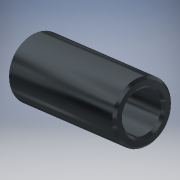
# Autodesk Inventor part: Component 31(Rod Axle)
Saved by Autodesk Inventor 2018 (Build 220112000, 112)
## iProperties
Created: 2023-04-01
Part Number: Component 31(Rod Axle)
Material: Generic
Document SubType Name: Modeling
Designer: Habib Mohamed
Density: 1 g/cm^3
Appearance: Iron Gray
Author: Habib Mohamed
Autodesk Inventor part; units mm, degrees
ref_plane "YZ Plane" through (0, 0, 0) normal (1, 0, 0) x (0, 1, 0)
ref_plane "XZ Plane" through (0, 0, 0) normal (0, 1, 0) x (-1, 0, 0)
ref_plane "XY Plane" through (0, 0, 0) normal (0, 0, 1) x (1, 0, 0)
sketch "Sketch1" plane through (0, 0, 0) normal (1, 0, 0) x (0, 1, 0)
  circle A0 centre (0, 0) radius 3
  circle A1 centre (0, 0) radius 2
  dimension "d0" = 6
  dimension "d1" = 4
  constraints: 2 centre point, 2 coincident
  measures "d0" diameter of A0
  measures "d1" diameter of A1
extrude "Extrusion1" add sketch "Sketch1" along normal blind 13
chamfer "Chamfer1" distance 0.25 angle 45 4 edges at (13, -3, 0) (13, -2, 0) (0, -2, 0) (0, -3, 0)
body "Solid1"
